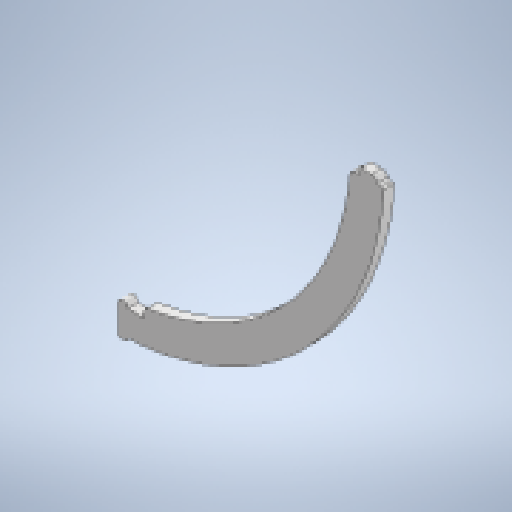
# Autodesk Inventor part: shim_cartridge_V3
Saved by Autodesk Inventor 2024.3 (Build 283343000, 343)
## iProperties
Created: 2024-04-08
Part Number: shim_cartridge_V3
Material: Generic
Document SubType Name: Modeling
Designer: Joshua Harper
Density: 1 g/cm^3
Appearance: Default
Author: Joshua Harper
Autodesk Inventor part; units mm, degrees
ref_plane "YZ Plane" through (0, 0, 0) normal (1, 0, 0) x (0, 1, 0)
ref_plane "XZ Plane" through (0, 0, 0) normal (0, 1, 0) x (-1, 0, 0)
ref_plane "XY Plane" through (0, 0, 0) normal (0, 0, 1) x (1, 0, 0)
sketch "Sketch1" plane through (0, 0, 0) normal (0, 0, 1) x (1, 0, 0)
  arc A0 (2, -80.9753) -> (80.9861, -1.5) centre (0, 0) ccw
  arc A1 (10, -70.2922) -> (70.9842, -1.5) centre (0, 0) ccw
  line L0 (10, -73.0753) -> (10, -70.2922)
  line L1 (70.9842, -1.5) -> (80.9861, -1.5)
  line L2 (0, 0) -> (0, 0) construction
  line L3 (10, -73.0753) -> (2, -73.0753)
  line L4 (2, -73.0753) -> (2, -80.9753)
  point P0 (75.9851, -1.5)
  dimension "d0" = 162
  dimension "d1" = 142
  dimension "d12" = 8
  dimension "d13" = 2
  dimension "d14" = 7.9
  dimension "d23" = 1.5
  constraints: 10 end point, 5 coincident, 4 point on circle, 2 centre point, 2 horizontal, 2 vertical, 1 midpoint, 1 perpendicular
  measures "d0" diameter of A0
  measures "d1" diameter of A1
  measures "d12" distance of L0.start L3.end
  measures "d13" distance between parallel lines of L4 L2
  measures "d14" distance of L4.end L3.end
  measures "d23" distance from line of L1 L2.end
extrude "Extrusion1" add sketch "Sketch1" along normal blind 3
sketch "Sketch3" plane through (0, 0, 3) normal (0, 0, 1) x (1, 0, 0)
  line L0 (10, -73.0753) -> (2, -73.0753) projected
  circle A0 centre (3.5, -73.0753) radius 1.5
  line L1 (2, -73.0753) -> (2, -80.9753) construction
  line L2 (2, -77.0253) -> (11.8753, -77.0253) construction
  ellipse E0 centre (3.5, -81.0253) end of major axis (5, -81.0253) minor radius 0.75
  point P0 (0, 0)
  point P1 (5, -73.0753)
  dimension "d15" = 3
  dimension "d16" = 1.5
  dimension "d20" = 0.75
  dimension "d21" = 1.5
  dimension "d22" = 4
  constraints: 2 centre point, 2 end point, 1 horizontal, 1 midpoint, 1 point on line, 1 vertical alignment, 1 other
  measures "d15" diameter of A0
  measures "d16" distance of A0.centre L0.end
  measures "d22" distance from line of E0.centre L2
extrude "Extrusion3" add sketch "Sketch3" against normal up to surface (3 mm away) contours L0 A0 | E0 picked at (3.784, -72.1991)
fillet "Fillet1" radius 1 2 edges at (10, -73.0753, 1.5) (10, -70.2922, 1.5)
sketch "Sketch4" plane through (0, 0, 3) normal (0, 0, 1) x (1, 0, 0)
  line L0 (80.9861, -1.5) -> (70.9842, -1.5) projected
  line L1 (80.9861, -1.5) -> (78.9861, -1.5)
  line L2 (78.9861, -4) -> (80.9012, -4)
  arc A0 (4.9576, -80.8481) -> (80.9861, -1.5) centre (0, 0) ccw projected
  arc A1 (80.9012, -4) -> (80.9861, -1.5) centre (0, 0) ccw
  line L3 (78.9861, -1.5) -> (78.9861, -4)
  line L4 (74.2542, -1.5) -> (70.9842, -1.5)
  arc A2 (10.8472, -70.1665) -> (70.9842, -1.5) centre (0, 0) ccw projected
  arc A3 (70.8727, -4.25) -> (70.9842, -1.5) centre (0, 0) ccw
  line L5 (70.8727, -4.25) -> (74.2542, -4.25)
  line L6 (74.2542, -4.25) -> (74.2542, -1.5)
  point P0 (10, -70.2922)
  dimension "d25" = 2.5
  dimension "d30" = 2
  dimension "d31" = 2.75
  dimension "d32" = 3.27
  constraints: 12 end point, 6 point on circle, 2 centre point, 2 concentric, 2 horizontal, 2 point on line, 1 collinear, 1 perpendicular, 1 vertical
  measures "d25" distance between parallel lines of L2 L0
  measures "d30" distance of L0.start L1.end
  measures "d31" distance between parallel lines of L0 L5
  measures "d32" distance of L0.end L4.start
extrude "Extrusion4" cut sketch "Sketch4" against normal blind 10
fillet "Fillet3" radius 0.75 3 edges at (70.8727, -4.25, 1.5) (74.2542, -4.25, 1.5) (78.9861, -4, 1.5)
fillet "Fillet4" radius 2 1 edges at (78.9861, -1.5, 1.5)
fillet "Fillet5" radius 0.5 1 edges at (74.2542, -1.5, 1.5)
equation "\"d16\" = 0.5 * d15"
body "Solid1"
